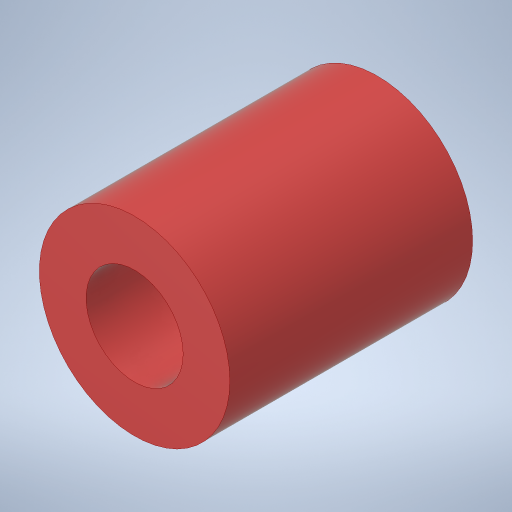
# Autodesk Inventor part: EL2-GB-009Spacer
Saved by Autodesk Inventor 2023.4 (Build 274418000, 418)
## iProperties
RuleStatus: InUse
Created: 2025-01-18
Part Number: EL2-GB-009Spacer
Material: ABS Plastic
Document SubType Name: Modeling
Designer: mavericks
Density: 1.06 g/cm^3
Appearance: Smooth - Red
AfterDocNew0: SHOW
AfterDocNew1: DISABLE SHOW
AfterDocNew2: size
AfterDocNew3: shaft size
AfterDocNew4: thunder
AfterAnyParamChange0: size
AfterAnyParamChange1: shaft size
AfterAnyParamChange2: thunder
AfterAnyUserParamChange0: size
AfterAnyUserParamChange1: thunder
AfterAnyUserParamChange2: shaft size
Author: mavericks
Autodesk Inventor part; units mm, degrees
ref_plane "YZ Plane" through (0, 0, 0) normal (1, 0, 0) x (0, 1, 0)
ref_plane "XZ Plane" through (0, 0, 0) normal (0, 1, 0) x (-1, 0, 0)
ref_plane "XY Plane" through (0, 0, 0) normal (0, 0, 1) x (1, 0, 0)
sketch "Sketch1" plane through (0, 0, 0) normal (0, 0, 1) x (1, 0, 0)
  circle A0 centre (0, 0) radius 3.302
  circle A1 centre (0, 0) radius 6.477
  dimension "Hex" = 6.604
  dimension "Thickness" = 3.175
  constraints: 2 centre point, 2 coincident
  measures "Hex" diameter of A0
  measures "Thickness" radial gap between concentric circles of A1 A0
extrude "Extrusion1" add sketch "Sketch1" along normal mid plane 16.51
equation "\"Tolerance_H\" = 0.3"
equation "\"Size\" = 12.7"
equation "\"Length\" = 30.2768"
equation "\"Tolerance_L\" = 0.508"
equation "\"Final_Metric\" = Hex"
equation "\"Thunder\" = 13.7541"
body "Solid1"
